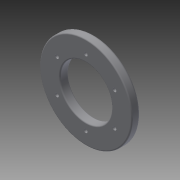
# Autodesk Inventor part: encoder_wheel
Saved by Autodesk Inventor 2014 SP1 (Build 180222100, 222)
## iProperties
Created: 2014-09-21
Part Number: encoder_wheel
Material: Générique
Document SubType Name: Modeling
Designer: astralien3000
Density: 1 g/cm^3
Appearance: Par défaut
d0: 75,000 mm
d1: 42,000 mm
d2: 7,000 mm
d3: 0,00 deg
d4: 2,000 mm
d5: 1,000 mm
d6: 1,000 mm
d7: 27,000 mm
d8: 3,000 mm
d9: 6,000 nd
d14: 0,00 deg
d11: 360,00 deg
Author: astralien3000
Autodesk Inventor part; units mm, degrees
ref_plane "YZ Plane" through (0, 0, 0) normal (1, 0, 0) x (0, 1, 0)
ref_plane "XZ Plane" through (0, 0, 0) normal (0, 1, 0) x (-1, 0, 0)
ref_plane "XY Plane" through (0, 0, 0) normal (0, 0, 1) x (1, 0, 0)
sketch "Esquisse1" plane through (0, 0, 0) normal (0, 1, 0) x (-1, 0, 0)
  circle A0 centre (0, 0) radius 37.5
  circle A1 centre (0, 0) radius 21
  dimension "d0" = 75
  dimension "d1" = 42
  constraints: 2 centre point, 2 coincident
  measures "d0" diameter of A0
  measures "d1" diameter of A1
extrude "Extrusion1" add sketch "Esquisse1" along normal blind 7
fillet "Congé1" radius 2 1 edges at (37.5, 7, 0)
fillet "Congé2" radius 1 1 edges at (21, 7, 0)
fillet "Congé3" radius 1 2 edges at (37.5, 0, 0) (21, 0, 0)
sketch "Esquisse2" plane through (0, 0, 0) normal (0, -1, 0) x (1, 0, 0)
  circle A0 centre (0, 0) radius 36.5 projected
  circle A1 centre (0, 0) radius 22 projected
  line L0 (0, 0) -> (0, 36.5) construction
  circle A2 centre (0, 27) radius 1.5
  circle A3 centre (-23.3827, 13.5) radius 1.5
  circle A4 centre (-23.3827, -13.5) radius 1.5
  circle A5 centre (0, -27) radius 1.5
  circle A6 centre (23.3827, -13.5) radius 1.5
  circle A7 centre (23.3827, 13.5) radius 1.5
  dimension "d7" = 27
  dimension "d8" = 3
  dimension "d11" = 360
  constraints: 6 centre point, 2 end point, 1 point on line, 1 vertical, 1 vertical alignment, 14 other
  measures "d7" distance of point (0, 0) A2.centre
  measures "d8" diameter of A2
extrude "Extrusion2" cut sketch "Esquisse2" against normal through all contours A2 | A3 | A4 | A5 | A6 | A7
